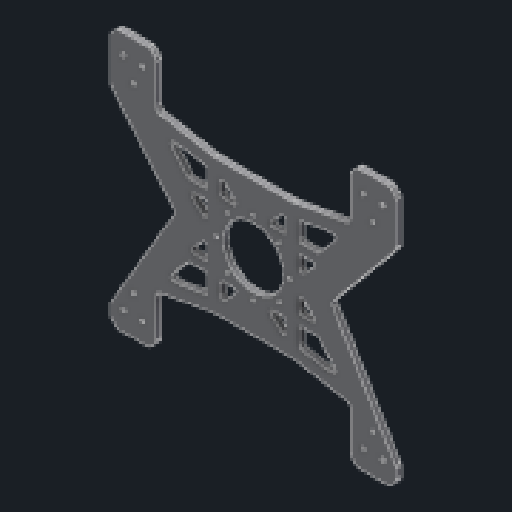
# Autodesk Inventor part: Root
Saved by Autodesk Inventor 2025.2 (Build 292293000, 293)
## iProperties
Created: 2020-05-07
Part Number: Root
Material: Generic
Document SubType Name: Sheet Metal
Designer: valer
Density: 1 g/cm^3
Sheet Metal Rule: Default
Appearance: Default
Author: valer
Autodesk Inventor part; units mm, degrees
ref_plane "YZ Plane" through (0, 0, 0) normal (1, 0, 0) x (0, 1, 0)
ref_plane "XZ Plane" through (0, 0, 0) normal (0, 1, 0) x (-1, 0, 0)
ref_plane "XY Plane" through (0, 0, 0) normal (0, 0, 1) x (1, 0, 0)
sketch "Base" plane through (0, 0, 0) normal (0, 0, 1) x (1, 0, 0)
  circle A0 centre (-56.25, 0) radius 2.75 construction
  circle A1 centre (0, -56.25) radius 2.75 construction
  circle A2 centre (0, 56.25) radius 2.75 construction
  circle A3 centre (39.7748, -39.7748) radius 2.75 construction
  circle A4 centre (-39.7748, 39.7748) radius 2.75 construction
  circle A5 centre (-39.7748, -39.7748) radius 2.75 construction
  circle A6 centre (39.7748, 39.7748) radius 2.75 construction
  circle A7 centre (56.25, 0) radius 2.75 construction
  circle A8 centre (0, 0) radius 45 construction
  circle A9 centre (0, 0) radius 61
  line L0 (220, -134.8551) -> (220, 200) construction
  line L1 (220, 200) -> (-220, 200) construction
  line L2 (-220, 200) -> (-220, -170) construction
  line L3 (0, -280) -> (0, 280) construction
  line L4 (-308, 0) -> (308, 0) construction
  line L5 (-220, 200) -> (-150, 200)
  line L6 (-150, 200) -> (-150, 120)
  line L7 (-150, 120) -> (-220, 120)
  line L8 (-220, 120) -> (-220, 200)
  line L9 (60, -103.923) -> (-60, -103.923)
  line L10 (-60, -103.923) -> (-120, 0)
  line L11 (-120, 0) -> (-60, 103.923)
  line L12 (-60, 103.923) -> (60, 103.923)
  line L13 (60, 103.923) -> (120, 0)
  line L14 (120, 0) -> (60, -103.923)
  line L15 (-120, 0) -> (-220, 120)
  line L16 (-150, 120) -> (-60, 103.923) construction
  line L17 (220, 200) -> (150, 200)
  line L18 (150, 200) -> (150, 120)
  line L19 (150, 120) -> (220, 120)
  line L20 (220, 120) -> (220, 200)
  line L21 (120, 0) -> (220, 120)
  line L22 (150, 120) -> (60, 103.923) construction
  line L23 (-220, -200) -> (-150, -200)
  line L24 (-150, -200) -> (-150, -120)
  line L25 (-150, -120) -> (-220, -120)
  line L26 (-220, -120) -> (-220, -200)
  line L27 (-120, 0) -> (-220, -120)
  line L28 (-150, -120) -> (-60, -103.923) construction
  line L29 (220, -120) -> (220, -200)
  line L30 (220, -200) -> (150, -200)
  line L31 (150, -200) -> (150, -120)
  line L32 (150, -120) -> (220, -120)
  line L33 (120, 0) -> (220, -120)
  line L34 (150, -120) -> (60, -103.923) construction
  circle A10 centre (0, 0) radius 46.5
  circle A11 centre (-56.25, 0) radius 2.25
  circle A12 centre (-39.7748, -39.7748) radius 2.25
  circle A13 centre (0, -56.25) radius 2.25
  circle A14 centre (39.7748, -39.7748) radius 2.25
  circle A15 centre (56.25, 0) radius 2.25
  circle A16 centre (39.7748, 39.7748) radius 2.25
  circle A17 centre (0, 56.25) radius 2.25
  circle A18 centre (-39.7748, 39.7748) radius 2.25
  line L35 (-150, 200) -> (-60, 103.923)
  line L36 (60, 103.923) -> (150, 200)
  line L37 (-150, -200) -> (-60, -103.923)
  line L38 (60, -103.923) -> (150, -200)
  point P0 (0, 0)
  dimension "d85" = 200
  dimension "d88" = 120
  dimension "d89" = 80
  dimension "d90" = 70
  dimension "d91" = 1.5
  dimension "d92" = 4.5
  dimension "d112" = 440
  measures "d85" distance between parallel lines of L1 L4
  measures "d88" distance of L9.start L9.end
  measures "d89" distance between parallel lines of L1 L7
  measures "d90" distance between parallel lines of L6 L8
  measures "d91" radial gap between concentric circles of A10 A8
  measures "d92" diameter of A11
  measures "d112" distance between parallel lines of L0 L2
extrude "Plate1" add sketch "Base" against normal blind 8.4667 contours A9 | L5 L6 L7 L8 | L35 L11 L15 L7 L6 | L12 L13 L14 L9 L10 L11 | L10 L37 L24 L25 L27 | L36 L18 L19 L21 L13 | L25 L24 L23 L26 | L33 L32 L31 L38 L14 | L17 L20 L19 L18 | L29 L30 L31 L32
sketch "LegMountHoles" plane through (0, 0, -8.4667) normal (0, 0, -1) x (-1, 0, 0)
  line L0 (-120, 0) -> (-220, 120) construction
  line L1 (-75.0601, 120) -> (-220, 120) construction
  line L2 (-220, 200) -> (-150, 200) construction
  line L3 (-185, 200) -> (-185, 120) construction
  line L4 (-170, 170) -> (-200, 170) construction
  circle A0 centre (-170, 170) radius 3
  circle A1 centre (-200, 170) radius 3
  circle A2 centre (-185, 140) radius 3
  line L5 (308, 0) -> (-308, 0) construction
  line L6 (0, -280) -> (0, 280) construction
  circle A3 centre (170, 170) radius 3
  circle A4 centre (200, 170) radius 3
  circle A5 centre (185, 140) radius 3
  circle A6 centre (-170, -170) radius 3
  circle A7 centre (-200, -170) radius 3
  circle A8 centre (-185, -140) radius 3
  circle A9 centre (170, -170) radius 3
  circle A10 centre (200, -170) radius 3
  circle A11 centre (185, -140) radius 3
  line L7 (-150, 200) -> (-60, 103.923) projected
  line L8 (-220, 120) -> (-220, 200) projected
  point P0 (0, 0)
  point P1 (-185, 170)
  dimension "d93" = 6
  dimension "d94" = 30
  dimension "d95" = 30
  dimension "d96" = 30
  constraints: 12 centre point, 9 symmetric about line, 6 end point, 4 point on line, 2 coincident, 2 equal radius, 2 horizontal, 2 midpoint, 2 perpendicular, 9 other
  measures "d93" diameter of A0
  measures "d94" distance of L4.start L4.end
  measures "d95" distance from line of L4 A2.centre
  measures "d96" distance between parallel lines of L2 L4
extrude "LegMountHolesFeature" cut sketch "LegMountHoles" against normal blind 8.4667
sketch "StructureHoles" plane through (0, 0, -8.4667) normal (0, 0, -1) x (-1, 0, 0)
  line L0 (70.4497, 85.8236) -> (97.321, 114.5093)
  line L1 (97.321, 114.5093) -> (149.3544, 114.5093)
  line L2 (149.3544, 114.5093) -> (100.4497, 55.8236)
  line L3 (100.4497, 55.8236) -> (70.4497, 55.8236)
  line L4 (70.4497, 55.8236) -> (70.4497, 85.8236)
  line L5 (220, 120) -> (120, 0) construction
  line L6 (150, 200) -> (220, 200) projected
  line L7 (-60, 103.923) -> (60, 103.923) projected
  line L8 (60, 103.923) -> (120, 0) construction
  line L9 (50.4497, 85.8236) -> (50.4497, 55.8236)
  line L10 (50.4497, 55.8236) -> (20.4497, 55.8236)
  line L11 (20.4497, 55.8236) -> (50.4497, 85.8236)
  line L12 (70.4497, 85.8236) -> (50.4497, 85.8236) construction
  line L13 (308, 0) -> (-308, 0) construction
  line L14 (0, -280) -> (0, 280) construction
  line L15 (-70.4497, 85.8236) -> (-97.321, 114.5093)
  line L16 (-97.321, 114.5093) -> (-149.3544, 114.5093)
  line L17 (-149.3544, 114.5093) -> (-100.4497, 55.8236)
  line L18 (-100.4497, 55.8236) -> (-70.4497, 55.8236)
  line L19 (-70.4497, 55.8236) -> (-70.4497, 85.8236)
  line L20 (-50.4497, 85.8236) -> (-50.4497, 55.8236)
  line L21 (-50.4497, 55.8236) -> (-20.4497, 55.8236)
  line L22 (-20.4497, 55.8236) -> (-50.4497, 85.8236)
  line L23 (70.4497, -85.8236) -> (97.321, -114.5093)
  line L24 (97.321, -114.5093) -> (149.3544, -114.5093)
  line L25 (149.3544, -114.5093) -> (100.4497, -55.8236)
  line L26 (100.4497, -55.8236) -> (70.4497, -55.8236)
  line L27 (70.4497, -55.8236) -> (70.4497, -85.8236)
  line L28 (50.4497, -85.8236) -> (50.4497, -55.8236)
  line L29 (50.4497, -55.8236) -> (20.4497, -55.8236)
  line L30 (20.4497, -55.8236) -> (50.4497, -85.8236)
  line L31 (-149.3544, -114.5093) -> (-100.4497, -55.8236)
  line L32 (-97.321, -114.5093) -> (-149.3544, -114.5093)
  line L33 (-70.4497, -85.8236) -> (-97.321, -114.5093)
  line L34 (-70.4497, -55.8236) -> (-70.4497, -85.8236)
  line L35 (-100.4497, -55.8236) -> (-70.4497, -55.8236)
  line L36 (-50.4497, -85.8236) -> (-50.4497, -55.8236)
  line L37 (-20.4497, -55.8236) -> (-50.4497, -85.8236)
  line L38 (-50.4497, -55.8236) -> (-20.4497, -55.8236)
  line L39 (100.4497, 40.8236) -> (70.4497, 10.8236)
  line L40 (70.4497, 10.8236) -> (70.4497, 40.8236)
  line L41 (70.4497, 40.8236) -> (100.4497, 40.8236)
  line L42 (100.4497, 55.8236) -> (100.4497, 40.8236) construction
  line L43 (100.4497, -40.8236) -> (70.4497, -10.8236)
  line L44 (70.4497, -10.8236) -> (70.4497, -40.8236)
  line L45 (70.4497, -40.8236) -> (100.4497, -40.8236)
  line L46 (-100.4497, 40.8236) -> (-70.4497, 10.8236)
  line L47 (-70.4497, 10.8236) -> (-70.4497, 40.8236)
  line L48 (-70.4497, 40.8236) -> (-100.4497, 40.8236)
  line L49 (-100.4497, -40.8236) -> (-70.4497, -10.8236)
  line L50 (-70.4497, -40.8236) -> (-100.4497, -40.8236)
  line L51 (-70.4497, -10.8236) -> (-70.4497, -40.8236)
  line L52 (60, 103.923) -> (150, 200) projected
  point P0 (0, 0)
  point P1 (85.4497, 40.8236)
  dimension "d101" = 30
  dimension "d102" = 30
  dimension "d103" = 20
  dimension "d106" = 15
  dimension "d113" = 20
  dimension "d114" = 52.0335
  constraints: 94 end point, 33 symmetric about line, 5 parallel, 4 perpendicular, 2 collinear, 2 equal length, 1 horizontal, 1 midpoint, 1 point on line, 1 vertical
  measures "d101" distance of L3.end L0.start
  measures "d102" distance of L2.end L3.end
  measures "d103" distance of L0.start L9.start
  measures "d106" distance from line of point (85.45, 40.824) L3
  measures "d113" distance between parallel lines of L52 L0
  measures "d114" distance of L0.end L1.end
extrude "StructureHolesFeature" cut sketch "StructureHoles" against normal blind 8.4667
fillet "InsideFilletsFeature" radius 4 44 edges at (-149.3544, 114.5093, -4.2333) (-97.321, 114.5093, -4.2333) (-70.4497, 85.8236, -4.2333) (-70.4497, 55.8236, -4.2333) (-100.4497, 55.8236, -4.2333) (97.321, 114.5093, -4.2333) (149.3544, 114.5093, -4.2333) (100.4497, 55.8236, -4.2333) (70.4497, 85.8236, -4.2333) (70.4497, 55.8236, -4.2333) (50.4497, 55.8236, -4.2333) (50.4497, 85.8236, -4.2333) (20.4497, 55.8236, -4.2333) (-50.4497, 85.8236, -4.2333) (-20.4497, 55.8236, -4.2333) (-50.4497, 55.8236, -4.2333) (-70.4497, 40.8236, -4.2333) (-100.4497, 40.8236, -4.2333) (-70.4497, 10.8236, -4.2333) (100.4497, 40.8236, -4.2333) (70.4497, 40.8236, -4.2333) (70.4497, 10.8236, -4.2333) (70.4497, -10.8236, -4.2333) (100.4497, -40.8236, -4.2333) (70.4497, -40.8236, -4.2333) (-100.4497, -40.8236, -4.2333) (-70.4497, -40.8236, -4.2333) (-70.4497, -10.8236, -4.2333) (-20.4497, -55.8236, -4.2333) (-50.4497, -85.8236, -4.2333) (-50.4497, -55.8236, -4.2333) (50.4497, -85.8236, -4.2333) (20.4497, -55.8236, -4.2333) (50.4497, -55.8236, -4.2333) (-149.3544, -114.5093, -4.2333) (-100.4497, -55.8236, -4.2333) (-70.4497, -55.8236, -4.2333) (-70.4497, -85.8236, -4.2333) (70.4497, -55.8236, -4.2333) (70.4497, -85.8236, -4.2333) (97.321, -114.5093, -4.2333) (149.3544, -114.5093, -4.2333) (100.4497, -55.8236, -4.2333) (-97.321, -114.5093, -4.2333)
chamfer "OutsideChamfersFeature" distance 10 angle 45 8 edges at (-220, -200, -4.2333) (-150, -200, -4.2333) (150, -200, -4.2333) (220, -200, -4.2333) (-220, 200, -4.2333) (-150, 200, -4.2333) (150, 200, -4.2333) (220, 200, -4.2333)
fillet "OutsideFilletsFeature" radius 8 25 edges at (60, 103.923, -4.2333) (160, 200, -4.2333) (210, 200, -4.2333) (220, 190, -4.2333) (220, 120, -4.2333) (120, 0, -4.2333) (220, -120, -4.2333) (220, -190, -4.2333) (210, -200, -4.2333) (160, -200, -4.2333) (60, -103.923, -4.2333) (-60, -103.923, -4.2333) (-160, -200, -4.2333) (-210, -200, -4.2333) (-220, -190, -4.2333) (-120, 0, -4.2333) (-220, 120, -4.2333) (-220, 190, -4.2333) (-210, 200, -4.2333) (-160, 200, -4.2333) (-60, 103.923, -4.2333) (-143.1635, 192.7019, -4.2333) (143.1635, 192.7019, -4.2333) (143.1635, -192.7019, -4.2333) (-143.1635, -192.7019, -4.2333)
equation "\"d97\" = Thickness"
equation "\"d104\" = Thickness"
equation "\"d33\" = Thickness"
equation "\"BendRadius\" = Thickness"
equation "\"BendReliefWidth\" = Thickness"
equation "\"BendReliefDepth\" = 0.5 * Thickness"
equation "\"CornerReliefSize\" = 4 * Thickness"
equation "\"MinimumRemnant\" = 2 * Thickness"
equation "\"TransitionRadius\" = BendRadius"
equation "\"JacobiRadiusSize\" = BendRadius"
equation "\"GapSize\" = Thickness"
equation "\"Thickness\" = 8.466667"
body "Solid1"
